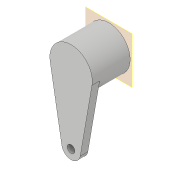
# Autodesk Inventor part: 20_Cube_Insert_Z-focus_Single_LED_arm
Saved by Autodesk Inventor 2019.4 (Build 234330000, 330)
## iProperties
Created: 2021-03-18
Part Number: 20_Cube_Insert_Z-focus_Single_LED_arm
Material: Generic
Document SubType Name: Modeling
Designer: diederichbenedict
Density: 1 g/cm^3
Appearance: Default
Author: diederichbenedict
Autodesk Inventor part; units mm, degrees
ref_plane "YZ Plane" through (0, 0, 0) normal (1, 0, 0) x (0, 1, 0)
ref_plane "XZ Plane" through (0, 0, 0) normal (0, 1, 0) x (-1, 0, 0)
ref_plane "XY Plane" through (0, 0, 0) normal (0, 0, 1) x (1, 0, 0)
ref_plane "Work Plane1" through (0, 0, 0) normal (0, 0, 1) x (1, 0, 0)
sketch "Sketch1" plane through (0, 0, 0) normal (0, 0, 1) x (1, 0, 0)
  circle A0 centre (0, 14.168) radius 14 projected
  circle A1 centre (8, 14.168) radius 2.45
  circle A2 centre (-8, 14.168) radius 2.45
  circle A3 centre (0, 14.168) radius 14
  circle A4 centre (0, 6.168) radius 2.45
  circle A5 centre (0, 22.168) radius 2.45
  point P0 (0, 0)
  dimension "d0" = 4.9
  dimension "d1" = 4.9
  dimension "d2" = 8
  dimension "d3" = 8
  dimension "d9" = 4.9
  dimension "d10" = 4.9
  dimension "d11" = 8
  dimension "d12" = 8
  constraints: 5 centre point, 1 coincident, 1 concentric
  measures "d0" diameter of A1
  measures "d1" diameter of A2
  measures "d2" distance of A0.centre A1.centre
  measures "d3" distance of A2.centre A0.centre
  measures "d9" diameter of A4
  measures "d10" diameter of A5
  measures "d11" distance of A0.centre A5.centre
  measures "d12" distance of A4.centre A0.centre
extrude "Extrusion1" add sketch "Sketch1" along normal blind 20
sketch "Sketch2" plane through (0, 14.168, 20) normal (0, 0, 1) x (1, 0, 0)
  circle A0 centre (-8, 0) radius 2.45 projected
  circle A1 centre (8, 0) radius 2.45 projected
  circle A2 centre (0, 0) radius 14 projected
  circle A3 centre (0, -45.639) radius 6.15 construction
  circle A4 centre (0, -45.639) radius 2.5
  line L0 (6.0583, -46.6969) -> (13.7914, -2.408)
  line L1 (-6.0583, -46.6969) -> (-13.7914, -2.408)
  circle A5 centre (0, 0) radius 14 projected
  arc A6 (-6.0583, -46.6969) -> (6.0583, -46.6969) centre (0, -45.639) ccw
  point P0 (0, -14.168)
  dimension "d6" = 5
  constraints: 6 point on circle, 6 tangent, 4 end point, 2 centre point, 1 coincident
  measures "d6" diameter of A4
extrude "Extrusion2" add sketch "Sketch2" along normal blind 5 contours A0 | A1 | A2 | A2 L0 A6 L1
body "Solid1"
